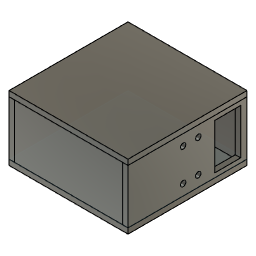
conntrol_box v1 (Autodesk Fusion 360 design; units mm, degrees)
Autodesk Fusion 360 part; units mm, degrees
sketch "Sketch1" plane through (0, 0, 0) normal (0, 1, 0) x (1, 0, 0)
  line L0 (0, 0) -> (110, 0)
  line L1 (110, 0) -> (110, 5)
  line L2 (110, 5) -> (0, 5)
  line L3 (0, 5) -> (0, 0)
  dimension "d1" = 110
  constraint coincident L0.start L3.end
  constraint horizontal L0
  constraint perpendicular L0 L1
  constraint perpendicular L1 L2
  constraint perpendicular L0 L3
  measures "d1" distance of L0.start L0.end
extrude "Extrude1" add sketch "Sketch1" along normal mid plane 110 makes body 1
sketch "Sketch2" plane through (0, 0, 0) normal (0, 0, 1) x (-1, 0, 0)
  line L0 (-110, 55) -> (-110, -55)
  line L1 (-110, -55) -> (0, -55)
  line L2 (0, -55) -> (0, 55)
  line L3 (0, 55) -> (-110, 55)
  line L4 (0, -55) -> (-5.0003, -55)
  line L5 (-5.0003, -55) -> (-5.0003, 55)
  line L6 (-5.0003, 55) -> (0, 55)
  line L7 (0, 55) -> (0, -55)
  constraint horizontal L4
  constraint vertical L5
  constraint horizontal L6
  constraint vertical L7
  constraint coincident L3 L5.end
  constraint coincident L1.end L2.start
extrude "Extrude2" add sketch "Sketch2" along normal blind 50 separate body contours L1 L2 L3 L4 L5 L6 L7 makes body 2
sketch "Sketch3" plane through (0, 0, 0) normal (0, 0, 1) x (1, 0, 0)
sketch "Sketch4" plane through (0, 0, 0) normal (0, 0, 1) x (-1, 0, 0)
  line L0 (-110, 55) -> (-110, -55)
  line L1 (-110, -55) -> (0, -55)
  line L2 (0, -55) -> (0, 55)
  line L3 (0, 55) -> (-110, 55)
  line L4 (-110, -55) -> (-105, -55)
  line L5 (-105, -55) -> (-105, 55)
  line L6 (-105, 55) -> (-110, 55)
  line L7 (-110, 55) -> (-110, -55)
  dimension "d6" = 5
  dimension "d7" = 110
  constraint horizontal L4
  constraint vertical L5
  constraint horizontal L6
  constraint vertical L7
  constraint coincident L0.end L1.start
  measures "d6" distance of L0.end L4.end
  measures "d7" distance of L0.end L0.start
extrude "Extrude3" add sketch "Sketch4" along normal blind 50 separate body contours L0 L1 L3 L4 L5 L6 L7 makes body 3
sketch "Sketch5" plane through (0, 0, 0) normal (0, 0, 1) x (-1, 0, 0)
  line L0 (-110, 55) -> (-110, -55)
  line L1 (-110, -55) -> (0, -55)
  line L2 (0, -55) -> (0, 55)
  line L3 (0, 55) -> (-110, 55)
sketch "Sketch6" plane through (0, 0, 0) normal (0, 0, 1) x (-1, 0, 0)
  line L0 (-105, 55) -> (-5, 55)
  line L1 (-5, 55) -> (-5, 50)
  line L2 (-5, 50) -> (-105, 50)
  line L3 (-105, 50) -> (-105, 55)
  constraint horizontal L0
  constraint vertical L1
  constraint horizontal L2
  constraint vertical L3
extrude "Extrude4" add sketch "Sketch6" along normal blind 50 separate body makes body 4
sketch "Sketch7" plane through (0, 0, 0) normal (0, 0, 1) x (1, 0, 0)
  line L0 (105, 55) -> (5, 55)
  line L1 (5, 55) -> (5, 50)
  line L2 (5, 50) -> (105, 50)
  line L3 (105, 50) -> (105, 55)
  constraint horizontal L0
  constraint vertical L1
  constraint horizontal L2
  constraint vertical L3
extrude "Extrude5" add sketch "Sketch7" along normal blind 50 separate body makes body 5
sketch "Sketch8" plane through (110, 0, 0) normal (1, 0, 0) x (0, 1, 0)
  line L0 (-55, 0) -> (55, 0)
  line L1 (55, 0) -> (55, 50)
  line L2 (55, 50) -> (-55, 50)
  line L3 (-55, 50) -> (-55, 0)
  line L4 (-55, 50) -> (55, 50)
  line L5 (55, 50) -> (55, 55)
  line L6 (55, 55) -> (-55, 55)
  line L7 (-55, 55) -> (-55, 50)
  constraint horizontal L4
  constraint vertical L5
  constraint horizontal L6
  constraint vertical L7
  constraint coincident L2.end L3.start
extrude "Extrude6" add sketch "Sketch8" against normal blind 110 separate body contours L2 L4 L5 L6 L7 makes body 6
sketch "Sketch9" plane through (110, 0, 0) normal (1, 0, 0) x (0, 1, 0)
  line L0 (-55, 0) -> (55, 0)
  line L1 (55, 0) -> (55, 50)
  line L2 (55, 50) -> (-55, 50)
  line L3 (-55, 50) -> (-55, 0)
  line L4 (49.2314, 3.9692) -> (25.2314, 3.9692)
  line L5 (25.2314, 3.9692) -> (25.2314, 45.9692)
  line L6 (25.2314, 45.9692) -> (49.2314, 45.9692)
  line L7 (49.2314, 45.9692) -> (49.2314, 3.9692)
  dimension "d16" = 24
  dimension "d17" = 42
  constraint horizontal L4
  constraint vertical L5
  constraint horizontal L6
  constraint vertical L7
  measures "d16" distance of L4.start L4.end
  measures "d17" distance of L4.start L6.end
extrude "Extrude7" cut sketch "Sketch9" against normal blind 15 contours L4 L5 L6 L7 bodies 3
sketch "Sketch10" plane through (110, 0, 0) normal (1, 0, 0) x (0, 1, 0)
  line L0 (25.2314, 3.9692) -> (25.2314, 45.9692)
  line L1 (25.2314, 45.9692) -> (49.2314, 45.9692)
  line L2 (49.2314, 45.9692) -> (49.2314, 3.9692)
  line L3 (49.2314, 3.9692) -> (25.2314, 3.9692)
  line L4 (-55, 0) -> (55, 0)
  line L5 (55, 0) -> (55, 50)
  line L6 (55, 50) -> (-55, 50)
  line L7 (-55, 50) -> (-55, 0)
  line L8 (10, 0) -> (10, 50)
  line L9 (10, 50) -> (10, 40)
  line L10 (10, 0) -> (10, 10)
  circle A0 centre (10, 10) radius 2.5
  circle A1 centre (10, 40) radius 2.5
  dimension "d20" = 5
  dimension "d21" = 5
  constraint coincident L4 L8.start
  constraint coincident L6 L8.end
  constraint perpendicular L6 L8
  constraint coincident L8 L9.end
  constraint perpendicular L4 L9
  constraint coincident L8 L10.end
  constraint coincident L10.end A0.centre
  constraint coincident L9.end A1.centre
  measures "d20" diameter of A0
  measures "d21" diameter of A1
hole "Hole1" at (110, 10, 40) direction (-1, 0, 0) diameter 5 depth 5 tip angle 118 bodies 3
hole "Hole2" at (110, 10, 10) direction (-1, 0, 0) diameter 5 depth 5 tip angle 118 bodies 3
sketch "Sketch11" plane through (110, 0, 0) normal (1, 0, 0) x (0, 1, 0)
  line L0 (10, 10) -> (-4, 10)
  line L1 (-4, 10) -> (-4, 40)
  line L2 (-4, 40) -> (10, 40)
  constraint horizontal L0
  constraint perpendicular L0 L1
  constraint perpendicular L1 L2
hole "Hole3" at (110, -4, 40) direction (-1, 0, 0) diameter 5 depth 5 tip angle 118 bodies 3
hole "Hole4" at (110, -4, 10) direction (-1, 0, 0) diameter 5 depth 5 tip angle 118 bodies 3
sketch "Sketch12" plane through (0, 0, 0) normal (-1, 0, 0) x (0, -1, 0)
  line L0 (-55, 0) -> (55, 0)
  line L1 (55, 0) -> (55, 50)
  line L2 (55, 50) -> (-55, 50)
  line L3 (-55, 50) -> (-55, 0)
  circle A0 centre (45, 5) radius 3
  dimension "d34" = 6
  measures "d34" diameter of A0
extrude "Extrude8" cut sketch "Sketch12" against normal blind 20 contours A0 bodies 2
copy_body "Body->Comp1" bodies 2 removing the originals makes body 7 in component "Component"
copy_body "Body->Comp2" bodies 6 removing the originals makes body 8 in component "Component'"
copy_body "Body->Comp3" bodies 5 removing the originals makes body 9 in component "Component''"
copy_body "Body->Comp4" bodies 4 removing the originals makes body 10 in component "Component'''"
copy_body "Body->Comp5" bodies 3 removing the originals makes body 11 in component "Component''''"
copy_body "Body->Comp6" bodies 1 removing the originals makes body 12 in component "Component'''''"
component "Component" placed x (1, 0, 0) y (0, 1, 0) z (0, 0, 1) at (0, 0, 0)
component "Component'" placed x (1, 0, 0) y (0, 1, 0) z (0, 0, 1) at (0, 0, 0)
component "Component''" placed x (1, 0, 0) y (0, 1, 0) z (0, 0, 1) at (0, 0, 0)
component "Component'''" placed x (1, 0, 0) y (0, 1, 0) z (0, 0, 1) at (0, 0, 0)
component "Component''''" placed x (1, 0, 0) y (0, 1, 0) z (0, 0, 1) at (0, 0, 0)
component "Component'''''" placed x (1, 0, 0) y (0, 1, 0) z (0, 0, 1) at (0, 0, 0)
